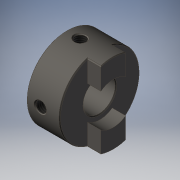
# Autodesk Inventor part: 60199320_2_20
Saved by Autodesk Inventor 2019 (Build 230136000, 136)
## iProperties
Created: 2024-03-16
Part Number: 60199320_2_20
Material: Generic
Catalog Web Link: www.cadenas.de
Description: na3_hzd_rf-Hub 3, Torsionally-Stiff Couplings HZD with Through Holes, Stainless, Set-screw style
Vendor: MAEDLER
Document SubType Name: Modeling
Designer: psAdmin
Manufacturer: MAEDLER
Mass: 36.0993 g
Surface Area: 91.8397 cm^2
Volume: 36.0993 cm^3
Density: 1 g/cm^3
Appearance: PSOLRGB-222-219-214
Category: PARTsolutions
Company: MAEDLER
Title: 60199320
Author: Cadenas PARTsolutions
Comments: Hub 3, Torsionally-Stiff Couplings HZD with Through Holes, Stainless, Set-screw style
PSOL_IDENT_0: {$CADENAS_DATA/23d-libs/maedler/antriebselemente/kupplungen/drehstarre_kupplungen/dr_k_hzd_m_db_rf/n
PSOL_IDENT_1: a3_hzd_rf.prj},172 {VTYP=3D},{NB=60199320_2_20},{LINA=60199320},{NN=na3_hzd_rf},{DATE=09.12.2023 00:
PSOL_IDENT_2: 25:54},{GEOMDATE=01.12.2023 07:25:45},{VERSION=},{LINEID=230},{WBVAR=BX1},{WBNUMERIC=BX1}  {NB=60199
PSOL_IDENT_3: 320_2_20},{LINA=60199320},{KT=DUMMY},{ARTNR=60199320},{WEBSHOP=Produktdetails / Katalogseite / Monta
PSOL_IDENT_4: geanleitung},{MATK=Edelstahl},{MAT=Naben aus Edelstahl rostfrei 1.4305 (V2A), Übertragungselement (K
PSOL_IDENT_5: reuzscheibe) aus schwarzem Polyacetal},{DM=30},{SBM=95},{B=20},{BMAX=25},{BX1=20.000},{L1=59.6},{L2=
PSOL_IDENT_6: 20.6},{L3=18.4},{D1=50.0},{MVW=±0.5},{MVR=±0.25},{VS=1375},{GEW=510},{ARTNR1=60125000},{GEW1=20.0},{
PSOL_IDENT_7: L4=20.6},{L5=29.00},{B1=15.45},{AB=42.65},{G=8},{AZ=2},{KB=16.6},{KB2=23.4},{KB3=22.0},{KB4=15.45},{
PSOL_IDENT_8: KTF=7.50},{KFT2=5.750},{KFT3=3.85},{KFT4=3.85},{FB=26},{TN=nabe3_kpl_hzd_rf_50.0_20},{CTN=84836080}
NB: 60199320_2_20
NN: na3_hzd_rf
NT: Hub 3, Torsionally-Stiff Couplings HZD with Through Holes, Stainless, Set-screw style
NBSYN: $ARTNR._2_$BX1.
LINA: 60199320
CATALOG: Mädler
ARTNR: 60199320
WEBSHOP: Produktdetails / Katalogseite / Montageanleitung
MATK: Edelstahl
MAT: Naben aus Edelstahl rostfrei 1.4305 (V2A), Übertragungselement (Kreuzscheibe) aus schwarzem Polyacetal
DM: 30
SBM: 95
B: 20
BMAX: 25
BX1: 20
L1: 59.6
L2: 20.6
L3: 18.4
D1: 50
MVW: ±0.5
MVR: ±0.25
VS: 1375
GEW: 510
ARTNR1: 60125000
GEW1: 20
L4: 20.6
L5: 29
B1: 15.45
AB: 42.65
G: 8
AZ: 2
KB: 16.6
KB2: 23.4
KB3: 22
KB4: 15.45
KTF: 7.5
KFT2: 5.75
KFT3: 3.85
KFT4: 3.85
FB: 26
TN: nabe3_kpl_hzd_rf_50.0_20
CTN: 84836080
SUPPLIER: MAEDLER
ARTICLENO: 60199320_2_20
BOMINFO: 60199320
CREATOR: CADENAS GmbH
Autodesk Inventor part; units mm, degrees
ref_plane "YZ Plane" through (0, 0, 0) normal (1, 0, 0) x (0, 1, 0)
ref_plane "XZ Plane" through (0, 0, 0) normal (0, 1, 0) x (-1, 0, 0)
ref_plane "XY Plane" through (0, 0, 0) normal (0, 0, 1) x (1, 0, 0)
sketch "Sketch_1" plane through (0, 0, 0) normal (0, 0, 1) x (1, 0, 0)
  line L0 (500, 0) -> (-500, 0)
  line L1 (-29.8, 24.6251) -> (-29.8, 10.3912)
  line L2 (-29.8, 10.3912) -> (-29.4887, 10)
  line L3 (-29.4887, 10) -> (-0.8, 10)
  line L4 (-0.8, 10) -> (-0.8, 24.6849)
  line L5 (-0.8, 24.6849) -> (-1.1882, 25)
  line L6 (-1.1882, 25) -> (-29.4692, 25)
  line L7 (-29.4692, 25) -> (-29.8, 24.6251)
  constraints: 16 end point
revolve "Revolution1" add sketch "Sketch_1" angle 360 about axis through (500, 0, 0) along (1, 0, 0)
sketch "Sketch_2" plane through (-0.8, 0, 0) normal (1, 0, 0) x (0, 0, -1)
  circle A0 centre (0, 0) radius 50
  line L0 (-7.725, -10.4558) -> (-7.725, -23.7766)
  arc A1 (-7.725, -23.7766) -> (7.725, -23.7766) centre (0, 0) ccw
  line L1 (7.725, -23.7766) -> (7.725, -10.4558)
  arc A2 (-7.725, -10.4558) -> (7.725, -10.4558) centre (0, 0) ccw
  arc A3 (7.725, 10.4558) -> (-7.725, 10.4558) centre (0, 0) ccw
  line L2 (7.725, 10.4558) -> (7.725, 23.7766)
  arc A4 (7.725, 23.7766) -> (-7.725, 23.7766) centre (0, 0) ccw
  line L3 (-7.725, 23.7766) -> (-7.725, 10.4558)
  constraints: 8 end point, 8 point on circle, 5 centre point
extrude "Extrusion1" cut sketch "Sketch_2" against normal blind 8.4
sketch "Sketch_4" plane through (0, 0, 0) normal (0, 0, 1) x (1, 0, 0)
  line L0 (-21.325, 25) -> (-21.325, 8.5)
  line L1 (-21.325, 8.5) -> (-25.325, 8.5)
  line L2 (-25.325, 8.5) -> (-24.6485, 9.1765)
  line L3 (-24.6485, 9.1765) -> (-24.6485, 24.3235)
  line L4 (-24.6485, 24.3235) -> (-25.325, 25)
  line L5 (-25.325, 25) -> (-21.325, 25)
  line L6 (-21.325, 25) -> (-21.325, 8.5)
  constraints: 14 end point
revolve "Revolution2" cut sketch "Sketch_4" angle 360 about axis through (-21.325, 25, 0) along (0, 1, 0)
thread "Thread1" size "M8x1.25" class "6H" standard "ISO Metric profile" full length
sketch "Sketch_5" plane through (0, 0, 0) normal (0, -1, 0) x (1, 0, 0)
  line L0 (-21.325, 25) -> (-21.325, 9)
  line L1 (-21.325, 9) -> (-25.325, 9)
  line L2 (-25.325, 9) -> (-24.6485, 9.6765)
  line L3 (-24.6485, 9.6765) -> (-24.6485, 24.3235)
  line L4 (-24.6485, 24.3235) -> (-25.325, 25)
  line L5 (-25.325, 25) -> (-21.325, 25)
  line L6 (-21.325, 25) -> (-21.325, 9)
  constraints: 14 end point
revolve "Revolution3" cut sketch "Sketch_5" angle 360 about axis through (-21.325, 0, 25) along (0, 0, 1)
thread "Thread2" size "M8x1.25" class "6H" standard "ISO Metric profile" length 14.647
chamfer "Chamfer1" distance 0.5 angle 45 6 edges at (-5.1941, -23.7766, -7.725) (-9.2, 0, -25) (-9.2, 0, 25) (-5.1941, 23.7766, -7.725) (-5.1941, -23.7766, 7.725) (-5.1941, 23.7766, 7.725)
chamfer "Chamfer2" distance 0.5 angle 45 1 edges at (-9.2, -10, 0)
ref_plane "center_XY" through (0, 0, 0) normal (1, 0, 0) x (0, 0, -1)
ref_plane "center_YZ" through (0, 0, 0) normal (0, 0, -1) x (0, 1, 0)
ref_plane "center_ZX" through (0, 0, 0) normal (0, 1, 0) x (1, 0, 0)
ref_plane "gew1_XY" through (-21.325, 25, 0) normal (0, 1, 0) x (1, 0, 0)
ref_plane "gew1_YZ" through (-21.325, 25, 0) normal (1, 0, 0) x (0, 0, -1)
ref_plane "gew1_ZX" through (-21.325, 25, 0) normal (0, 0, -1) x (0, 1, 0)
ref_plane "gew2_XY" through (-21.325, 0, 25) normal (0, 0, 1) x (1, 0, 0)
ref_plane "gew2_YZ" through (-21.325, 0, 25) normal (1, 0, 0) x (0, 1, 0)
ref_plane "gew2_ZX" through (-21.325, 0, 25) normal (0, 1, 0) x (0, 0, 1)
body "Solid1"
